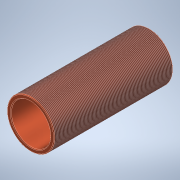
# Autodesk Inventor part: 4111_Bias_Coil_Layer2_MPSv2_v1
Saved by Autodesk Inventor 2021 (Build 250183000, 183)
## iProperties
Created: 2020-11-17
Part Number: 4111_Bias_Coil_Layer2_MPSv2_v1
Material: Copper
Document SubType Name: Modeling
Designer: Admin
Density: 8.94 g/cm^3
Appearance: Copper - Satin
Author: Admin
Autodesk Inventor part; units mm, degrees
ref_plane "YZ Plane" through (0, 0, 0) normal (1, 0, 0) x (0, 1, 0)
ref_plane "XZ Plane" through (0, 0, 0) normal (0, 1, 0) x (-1, 0, 0)
ref_plane "XY Plane" through (0, 0, 0) normal (0, 0, 1) x (1, 0, 0)
sketch "Sketch1" plane through (0, 0, 0) normal (0, 0, 1) x (1, 0, 0)
  circle A0 centre (0, 0) radius 35.835
  circle A1 centre (0, 0) radius 29.715
  dimension "d0" = 71.67
  dimension "d1" = 59.43
  constraints: 2 centre point, 2 coincident
  measures "d0" diameter of A0
  measures "d1" diameter of A1
extrude "Extrusion1" add sketch "Sketch1" along normal blind 180
thread "Thread1" size "M16x2" class "6g" standard "ANSI Metric M Profile" full length
fillet "Fillet1" radius 1 2 edges at (-35.835, 0, 180) (-29.715, 0, 180)
fillet "Fillet2" radius 1 2 edges at (-29.715, 0, 0) (-35.835, 0, 0)
body "Solid1"
